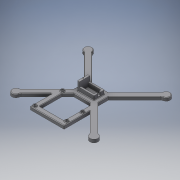
# Autodesk Inventor part: base
Saved by Autodesk Inventor 2020 (Build 240168000, 168)
## iProperties
Created: 2020-02-04
Part Number: base
Material: Generic
Document SubType Name: Modeling
Designer: Wes
Density: 1 g/cm^3
Appearance: Default
Author: Wes
Autodesk Inventor part; units mm, degrees
ref_plane "YZ Plane" through (0, 0, 0) normal (1, 0, 0) x (0, 1, 0)
ref_plane "XZ Plane" through (0, 0, 0) normal (0, 1, 0) x (-1, 0, 0)
ref_plane "XY Plane" through (0, 0, 0) normal (0, 0, 1) x (1, 0, 0)
sketch "Sketch1 - motor_fit" plane through (0, 0, 0) normal (0, 0, 1) x (1, 0, 0)
  line L0 (0, 29) -> (18.5, 29)
  line L1 (0, 14.5) -> (3, 14.5) construction
  line L2 (18.5, 14.5) -> (15.5, 14.5) construction
  line L3 (3, 3) -> (15.5, 3)
  line L4 (15.5, 3) -> (15.5, 26)
  line L5 (15.5, 26) -> (3, 26)
  line L6 (3, 26) -> (3, 3)
  line L7 (9.25, 3) -> (9.25, -0.5) construction
  line L8 (0, 29) -> (0, -0.5)
  line L9 (0, -0.5) -> (18.5, -0.5)
  line L10 (18.5, -0.5) -> (18.5, 29)
  dimension "d1" = 18.5
  dimension "d3" = 3
  dimension "d4" = 3
  dimension "d5" = 23
  dimension "d6" = 12.5
  dimension "d110" = 3.5
  dimension "d111" = 29.5
  constraints: 22 end point, 5 perpendicular, 3 horizontal, 2 vertical, 1 midpoint
  measures "d1" distance of L0.start L0.end
  measures "d3" distance of L1.start L1.end
  measures "d4" distance of L2.start L2.end
  measures "d5" distance of L3.end L4.end
  measures "d6" distance of L4.end L5.end
  measures "d110" distance of L7.start L7.end
  measures "d111" distance of L0.start L8.end
extrude "Extrusion1" add sketch "Sketch1 - motor_fit" along normal blind 7
sketch "Sketch2 motor_edge_mount" plane through (0, 0, 7) normal (0, 0, 1) x (1, 0, 0)
  line L0 (18.5, 3) -> (0, 3)
  line L1 (0, 3) -> (0, -0.5)
  line L2 (0, -0.5) -> (18.5, -0.5) projected
  line L3 (0, -0.5) -> (18.5, -0.5)
  line L4 (18.5, -0.5) -> (18.5, 3)
  constraints: 8 end point, 1 perpendicular, 1 vertical
extrude "Extrusion2" add sketch "Sketch2 motor_edge_mount" along normal blind 8.6
sketch "Sketch8 - motor_screw_hole" plane through (0, 0, 15.6) normal (0, 0, 1) x (1, 0, 0)
  line L0 (9.25, 3) -> (9.25, -1.7) construction
  line L1 (9.25, -1.7) -> (9.25, 0.3) construction
  circle A0 centre (9.25, 0.3) radius 0.9
  dimension "d105" = 4.7
  dimension "d106" = 2
  dimension "d107" = 1.8
  constraints: 4 end point, 1 centre point, 1 coincident, 1 point on line, 1 vertical
  measures "d105" distance of L0.start L0.end
  measures "d106" distance of L0.end L1.end
  measures "d107" diameter of A0
extrude "Extrusion8" cut sketch "Sketch8 - motor_screw_hole" against normal blind 5.6
sketch "Sketch3 - base_legs" plane through (0, 0, 0) normal (0, 0, -1) x (-1, 0, 0)
  line L0 (-9.25, 29) -> (-9.25, 36) construction
  line L1 (0, 14.5) -> (7, 14.5) construction
  line L2 (-18.5, 13) -> (-25.5, 13) construction
  line L3 (-25.5, 36) -> (7, 36)
  line L4 (-9.25, 0) -> (-9.25, -7) construction
  line L5 (-25.5, -7) -> (-25.5, 36)
  line L6 (-25.5, -7) -> (7, -7)
  line L7 (7, -7) -> (7, 36)
  line L8 (7, 29) -> (58.6188, 80.6188)
  line L9 (0, 36) -> (51.6188, 87.6188)
  line L10 (51.6188, 87.6188) -> (58.6188, 80.6188)
  line L11 (7, 0) -> (58.6188, -51.6188)
  line L12 (0, -7) -> (51.6188, -58.6188)
  line L13 (51.6188, -58.6188) -> (58.6188, -51.6188)
  circle A0 centre (55.1188, -55.1188) radius 7
  circle A1 centre (55.1188, 84.1188) radius 7
  line L14 (-18.5, -7) -> (-70.1188, -58.6188)
  line L15 (-25.5, 0) -> (-77.1188, -51.6188)
  line L16 (-77.1188, -51.6188) -> (-70.1188, -58.6188)
  circle A2 centre (-73.6188, -55.1188) radius 7
  line L17 (-25.5, 29) -> (-77.1188, 80.6188)
  line L18 (-77.1188, 80.6188) -> (-70.1188, 87.6188)
  line L19 (-70.1188, 87.6188) -> (-18.5, 36)
  line L20 (-18.5, 29) -> (-73.6188, 84.1188) construction
  circle A3 centre (-73.6188, 84.1188) radius 7
  point P0 (48.1188, -55.1188)
  point P1 (55.1188, -48.1188)
  point P2 (55.1188, 77.1188)
  point P3 (48.1188, 84.1188)
  point P4 (-73.6188, -48.1188)
  point P5 (-66.6188, -55.1188)
  point P6 (-66.6188, 84.1188)
  point P7 (-73.6188, 77.1188)
  dimension "d13" = 7
  dimension "d14" = 7
  dimension "d15" = 7
  dimension "d16" = 32.5
  dimension "d17" = 7
  dimension "d18" = 43
  dimension "d24" = 73
  dimension "d26" = 73
  dimension "d32" = 14
  dimension "d100" = 73
  dimension "d115" = 73
  dimension "d117" = 77.9497
  constraints: 42 end point, 8 point on line, 4 centre point, 4 horizontal, 4 midpoint, 4 perpendicular, 3 vertical, 1 coincident
  measures "d13" distance of L0.start L0.end
  measures "d14" distance of L1.start L1.end
  measures "d15" distance of L2.start L2.end
  measures "d16" distance of L3.start L3.end
  measures "d17" distance of L4.start L4.end
  measures "d18" distance of L5.start L3.start
  measures "d24" distance of L8.start L8.end
  measures "d26" distance of L11.start L11.end
  measures "d32" diameter of A0
  measures "d100" distance of L14.start L14.end
  measures "d115" distance of L18.end L19.end
  measures "d117" distance of L20.start L20.end
extrude "Extrusion3" add sketch "Sketch3 - base_legs" along normal blind 5.5
sketch "Sketch4 - wire_hole" plane through (0, 29, 7) normal (0, 1, 0) x (1, 0, 0)
  line L0 (9.25, 7) -> (9.25, 5) construction
  line L1 (6.75, 5) -> (11.75, 5)
  line L2 (11.75, 5) -> (11.75, 0)
  line L3 (6.75, 5) -> (6.75, 0)
  line L4 (6.75, 0) -> (11.75, 0)
  point P0 (0, 7)
  dimension "d38" = 2
  dimension "d39" = 5
  constraints: 10 end point, 3 vertical, 1 horizontal, 1 perpendicular
  measures "d38" distance of L0.start L0.end
  measures "d39" distance of L1.start L1.end
extrude "Extrusion4" cut sketch "Sketch4 - wire_hole" against normal blind 3
sketch "Sketch5 - arduino_base" plane through (0, 0, 0) normal (0, 0, 1) x (1, 0, 0)
  line L0 (25.5, 14.5) -> (32, 14.5) construction
  line L1 (33.3322, -21.8322) -> (40.3322, -14.8322) construction
  line L2 (32, -13.5) -> (32, -11.75) construction
  line L3 (32, -11.75) -> (32, 37.25) construction
  line L4 (32, 37.25) -> (75.35, 37.25) construction
  line L5 (75.35, 37.25) -> (80, 37.25) construction
  line L6 (32, 34.705) -> (47.15, 34.705) construction
  line L7 (47.15, 37.25) -> (47.15, 41.5) construction
  line L8 (47.15, 37.25) -> (47.15, 33) construction
  line L9 (29.5, 33) -> (38, 41.5)
  line L10 (80, 12.75) -> (75.75, 12.75) construction
  line L11 (80, 12.75) -> (84.25, 12.75) construction
  line L12 (75.75, 33) -> (29.5, 33)
  line L13 (84.25, 41.5) -> (38, 41.5)
  line L14 (61.125, -14.8322) -> (61.125, -10.5822) construction
  line L15 (61.125, -14.8322) -> (61.125, -19.0822) construction
  line L16 (75.75, 33) -> (75.75, -10.5822)
  line L17 (75.75, -10.5822) -> (36.0822, -10.5822)
  line L18 (84.25, 41.5) -> (84.25, -19.0822)
  line L19 (84.25, -19.0822) -> (44.5822, -19.0822)
  line L20 (44.5822, -19.0822) -> (36.0822, -10.5822)
  point P0 (0, 0)
  point P1 (80, -14.8322)
  dimension "d63" = 6.5
  dimension "d64" = 1.75
  dimension "d65" = 49
  dimension "d66" = 43.35
  dimension "d67" = 4.65
  dimension "d68" = 15.15
  dimension "d69" = 4.25
  dimension "d70" = 4.25
  dimension "d72" = 4.25
  dimension "d73" = 4.25
  dimension "d74" = 4.25
  dimension "d75" = 4.25
  constraints: 42 end point, 8 vertical, 6 horizontal, 4 perpendicular, 3 coincident, 2 point on line
  measures "d63" distance of L0.start L0.end
  measures "d64" distance of L2.start L2.end
  measures "d65" distance of L2.end L3.end
  measures "d66" distance of L4.start L4.end
  measures "d67" distance of L5.start L5.end
  measures "d68" distance of L6.start L6.end
  measures "d69" distance of L7.start L7.end
  measures "d70" distance of L7.start L8.end
  measures "d72" distance of L10.start L10.end
  measures "d73" distance of L10.start L11.end
  measures "d74" distance of L14.start L14.end
  measures "d75" distance of L14.start L15.end
extrude "Extrusion5" add sketch "Sketch5 - arduino_base" against normal blind 5.5
sketch "Sketch6 - arduino_raised" plane through (0, 0, 0) normal (0, 0, 1) x (1, 0, 0)
  line L0 (25.5, 14.5) -> (32, 14.5) construction
  line L1 (33.3322, -21.8322) -> (40.3322, -14.8322) construction
  line L2 (32, -13.5) -> (32, -11.75) construction
  line L3 (32, -11.75) -> (32, 37.25) construction
  line L4 (32, 37.25) -> (75.35, 37.25) construction
  line L5 (75.35, 37.25) -> (80, 37.25) construction
  line L6 (32, 34.705) -> (47.15, 34.705) construction
  line L7 (47.15, 37.25) -> (47.15, 41.5) construction
  line L8 (47.15, 37.25) -> (47.15, 33) construction
  circle A0 centre (32, -13.5) radius 2.75
  circle A1 centre (80, -14.8322) radius 2.75
  circle A2 centre (47.15, 37.25) radius 2.75
  circle A3 centre (75.35, 37.25) radius 2.75
  point P0 (0, 0)
  dimension "d78" = 6.5
  dimension "d79" = 1.75
  dimension "d80" = 49
  dimension "d81" = 43.35
  dimension "d82" = 4.65
  dimension "d83" = 15.15
  dimension "d84" = 4.25
  dimension "d85" = 4.25
  dimension "d90" = 5.5
  dimension "d93" = 5.5
  dimension "d94" = 5.5
  dimension "d97" = 5.5
  constraints: 18 end point, 7 coincident, 4 centre point, 4 vertical, 3 horizontal, 2 point on line, 1 perpendicular
  measures "d78" distance of L0.start L0.end
  measures "d79" distance of L2.start L3.start
  measures "d80" distance of L3.start L3.end
  measures "d81" distance of L4.start L4.end
  measures "d82" distance of L5.start L5.end
  measures "d83" distance of L6.start L6.end
  measures "d84" distance of L8.start L7.end
  measures "d85" distance of L8.start L8.end
  measures "d90" diameter of A0
  measures "d93" diameter of A1
  measures "d94" diameter of A2
  measures "d97" diameter of A3
extrude "Extrusion6" add sketch "Sketch6 - arduino_raised" along normal blind 1.8
sketch "Sketch7 - arduino_holes" plane through (0, 0, 1.8) normal (0, 0, 1) x (1, 0, 0)
  line L0 (30.5321, -19.0321) -> (37.5321, -12.0321) construction
  line L1 (37.5321, 41.0321) -> (30.5321, 48.0321) construction
  line L2 (25.5, 14.5) -> (32, 14.5) construction
  circle A0 centre (32, -13.5) radius 1.75
  line L3 (32, -11.75) -> (32, 37.25) construction
  line L4 (32, 37.25) -> (45.4, 37.25) construction
  line L5 (45.4, 37.25) -> (47.15, 37.25) construction
  circle A1 centre (47.15, 37.25) radius 1.75
  line L6 (48.9, 37.25) -> (73.6, 37.25) construction
  line L7 (73.6, 37.25) -> (75.35, 37.25) construction
  circle A2 centre (75.35, 37.25) radius 1.75
  line L8 (77.1, 37.25) -> (80, 37.25) construction
  line L9 (80, 37.25) -> (80, -13.15) construction
  line L10 (80, -13.15) -> (80, -14.9) construction
  circle A3 centre (80, -14.9) radius 1.75
  point P0 (0, 0)
  dimension "d47" = 3.5
  dimension "d55" = 3.5
  dimension "d58" = 3.5
  dimension "d45" = 6.5
  dimension "d52" = 49
  dimension "d53" = 13.4
  dimension "d54" = 1.75
  dimension "d56" = 24.7
  dimension "d57" = 1.75
  dimension "d59" = 2.9
  dimension "d60" = 50.4
  dimension "d61" = 1.75
  dimension "d62" = 3.5
  constraints: 22 end point, 5 horizontal, 3 coincident, 3 vertical, 2 horizontal alignment, 1 centre point, 1 perpendicular, 1 vertical alignment, 6 other
  measures "d45" distance of L2.start L2.end
  measures "d52" distance of L3.start L3.end
  measures "d53" distance of L3.end L4.end
  measures "d54" distance of L4.end L5.end
  measures "d56" distance of L6.start L6.end
  measures "d57" distance of L6.end L7.end
  measures "d59" distance of L8.start L8.end
  measures "d60" distance of L8.end L9.end
  measures "d61" distance of L9.end L10.end
  measures "d62" diameter of A3
extrude "Extrusion7" cut sketch "Sketch7 - arduino_holes" against normal blind 8.3
fillet "Fillet1 - feet_edges" radius 5 8 edges at (73.6188, -48.1188, -2.75) (-48.1188, 84.1188, -2.75) (66.6188, -55.1188, -2.75) (-48.1188, -55.1188, -2.75) (-55.1188, -48.1188, -2.75) (-55.1188, 77.1188, -2.75) (73.6188, 77.1188, -2.75) (66.6188, 84.1188, -2.75)
fillet "Fillet2 - other_smaller" radius 1 50 edges at (73.563, -47.7542, 0) (78.5685, -60.0685, 0) (66.2542, -55.063, 0) (41.9376, -30.4376, 0) (58.4787, -32.9787, 0) (55.9161, -10.5822, 0) (64.4161, -19.0822, 0) (84.25, 11.2089, 0) (75.75, 11.2089, 0) (52.625, 33, 0) (61.125, 41.5, 0) (-47.7542, 84.063, 0) (-60.0685, 89.0685, 0) (-55.063, 76.7542, 0) (-30.4376, 52.4376, 0) (-23.4376, 59.4376, 0) (9.25, 36, 0) (-7, 14.5, 0) (25.5, 14.5, 0) (30.7911, -5.2911, 0) (-55.063, -47.7542, 0) (-60.0685, -60.0685, 0) (-47.7542, -55.063, 0) (-23.4376, -30.4376, 0) (-30.4376, -23.4376, 0) (9.25, -7, 0) (18.5, -7, -2.75) (84.25, -19.0822, -2.75) (-7, 29, -2.75) (-7, 0, -2.75) (0, -7, -2.75) (0, 36, -2.75) (84.25, 41.5, -2.75) (25.5, 0, -2.75) (36.0822, -10.5822, -2.75) (75.75, 33, -2.75) (75.75, -10.5822, -2.75) (44.5822, -19.0822, -2.75) (18.5, 14.25, 0) (9.25, 29, 0) (0, 14.25, 0) (9.25, -0.5, 0) (18.5, 29, 3.5) (18.5, -0.5, 7.8) (0, 29, 3.5) (0, -0.5, 7.8) (44.4, 37.25, 0) (72.6, 37.25, 0) (77.25, -14.8322, 0) (29.25, -13.5, 0)
body "Solid1"
